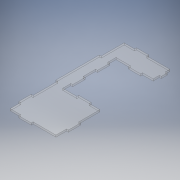
# Autodesk Inventor part: top
Saved by Autodesk Inventor 2017.2 (Build 212233000, 233)
## iProperties
Created: 2017-06-02
Part Number: top
Material: Polycarbonate, Clear
Document SubType Name: Modeling
Designer: SandeepSH
Density: 1.2 g/cm^3
Appearance: Polycarbonate - Clear
Author: SandeepSH
Autodesk Inventor part; units mm, degrees
ref_plane "YZ Plane" through (0, 0, 0) normal (1, 0, 0) x (0, 1, 0)
ref_plane "XZ Plane" through (0, 0, 0) normal (0, 1, 0) x (-1, 0, 0)
ref_plane "XY Plane" through (0, 0, 0) normal (0, 0, 1) x (1, 0, 0)
sketch "Sketch1" plane through (0, 0, 0) normal (0, 1, 0) x (-1, 0, 0)
  line L0 (-40, 95) -> (40, 95)
  line L1 (40, 95) -> (40, -95)
  line L2 (40, -95) -> (-40, -95)
  line L3 (-40, -95) -> (-40, 95)
  line L4 (-40, 95) -> (40, -95) construction
  line L5 (40, 95) -> (-40, -95) construction
  point P0 (0, 0)
  dimension "d0" = 80
  dimension "d1" = 190
  constraints: 12 end point, 2 midpoint, 2 parallel, 1 horizontal, 1 perpendicular
  measures "d0" distance of L1.end L2.end
  measures "d1" distance of L0.end L1.end
extrude "Extrusion1" add sketch "Sketch1" along normal blind 3
sketch "Sketch2" plane through (0, 3, 0) normal (0, 1, 0) x (1, 0, 0)
  line L0 (40, 95) -> (-40, 95) projected
  line L1 (-40, 95) -> (-37, 95)
  line L2 (-37, 95) -> (-37, 55)
  line L3 (-37, 55) -> (-40, 55)
  line L4 (-40, 55) -> (-40, 95)
  line L5 (-40, 95) -> (-40, -95) projected
  line L6 (-40, -95) -> (40, -95) projected
  line L7 (-37, 95) -> (-20, 95)
  line L8 (-20, 95) -> (-20, 92)
  line L9 (-20, 92) -> (-37, 92)
  line L10 (-37, 92) -> (-37, 95)
  line L11 (40, -95) -> (40, 95) projected
  line L12 (40, 95) -> (0, 95)
  line L13 (0, 95) -> (0, 92)
  line L14 (0, 92) -> (40, 92)
  line L15 (40, 92) -> (40, 95)
  line L16 (-40, -55) -> (-37, -55)
  line L17 (-37, -55) -> (-37, -15)
  line L18 (-37, -15) -> (-40, -15)
  line L19 (-40, -15) -> (-40, -55)
  line L20 (-40, -95) -> (-37, -95)
  line L21 (-37, -95) -> (-37, -75)
  line L22 (-37, -75) -> (-40, -75)
  line L23 (-40, -75) -> (-40, -95)
  line L24 (-37, -95) -> (-20, -95)
  line L25 (-20, -95) -> (-20, -92)
  line L26 (-20, -92) -> (-37, -92)
  line L27 (-37, -92) -> (-37, -95)
  line L28 (40, -95) -> (0, -95)
  line L29 (0, -95) -> (0, -92)
  line L30 (0, -92) -> (40, -92)
  line L31 (40, -92) -> (40, -95)
  line L32 (40, -18) -> (-20, -18)
  line L33 (-20, -18) -> (-20, 62)
  line L34 (-20, 62) -> (40, 62)
  line L35 (40, 62) -> (40, -18)
  line L36 (40, -92) -> (37, -92)
  line L37 (37, -92) -> (37, -75)
  line L38 (37, -75) -> (40, -75)
  line L39 (40, -75) -> (40, -92)
  line L40 (40, -18) -> (37, -18)
  line L41 (37, -18) -> (37, -55)
  line L42 (37, -55) -> (40, -55)
  line L43 (40, -55) -> (40, -18)
  line L44 (40, 92) -> (37, 92)
  line L45 (37, 92) -> (37, 85)
  line L46 (37, 85) -> (40, 85)
  line L47 (40, 85) -> (40, 92)
  line L48 (40, 62) -> (37, 62)
  line L49 (37, 62) -> (37, 75)
  line L50 (37, 75) -> (40, 75)
  line L51 (40, 75) -> (40, 62)
  line L52 (-20, -18) -> (-23, -18)
  line L53 (-23, -18) -> (-23, -8)
  line L54 (-23, -8) -> (-20, -8)
  line L55 (-20, -8) -> (-20, -18)
  line L56 (-20, 12) -> (-23, 12)
  line L57 (-23, 12) -> (-23, 32)
  line L58 (-23, 32) -> (-20, 32)
  line L59 (-20, 32) -> (-20, 12)
  line L60 (-20, 62) -> (-23, 62)
  line L61 (-23, 62) -> (-23, 52)
  line L62 (-23, 52) -> (-20, 52)
  line L63 (-20, 52) -> (-20, 62)
  line L64 (-23, -18) -> (0, -18)
  line L65 (0, -18) -> (0, -21)
  line L66 (0, -21) -> (-23, -21)
  line L67 (-23, -21) -> (-23, -18)
  line L68 (37, -18) -> (20, -18)
  line L69 (20, -18) -> (20, -21)
  line L70 (20, -21) -> (37, -21)
  line L71 (37, -21) -> (37, -18)
  line L72 (-23, 62) -> (0, 62)
  line L73 (0, 62) -> (0, 65)
  line L74 (0, 65) -> (-23, 65)
  line L75 (-23, 65) -> (-23, 62)
  line L76 (37, 62) -> (20, 62)
  line L77 (20, 62) -> (20, 65)
  line L78 (20, 65) -> (37, 65)
  line L79 (37, 65) -> (37, 62)
  point P0 (0, 0)
  dimension "d4" = 3
  dimension "d5" = 40
  dimension "d9" = 17
  dimension "d10" = 3
  dimension "d11" = 3
  dimension "d12" = 20
  dimension "d13" = 3
  dimension "d14" = 70
  dimension "d15" = 40
  dimension "d16" = 3
  dimension "d17" = 20
  dimension "d18" = 17
  dimension "d19" = 3
  dimension "d20" = 33
  dimension "d21" = 20
  dimension "d22" = 77
  dimension "d23" = 3
  dimension "d24" = 17
  dimension "d25" = 20
  dimension "d26" = 7
  dimension "d27" = 10
  dimension "d28" = 3
  dimension "d29" = 10
  dimension "d30" = 3
  dimension "d31" = 20
  dimension "d32" = 10
  dimension "d33" = 20
  dimension "d34" = 23
  dimension "d35" = 3
  dimension "d36" = 17
  dimension "d37" = 3
  dimension "d38" = 23
  dimension "d39" = 3
  dimension "d40" = 17
  dimension "d41" = 3
  constraints: 152 end point, 38 parallel, 19 horizontal, 19 perpendicular, 7 point on line
  measures "d4" distance of L2.end L3.end
  measures "d5" distance of L1.end L2.end
  measures "d9" distance of L8.end L9.end
  measures "d10" distance of L7.end L8.end
  measures "d11" distance of L13.end L12.end
  measures "d12" distance between parallel lines of L8 L13
  measures "d13" distance of L18.end L17.end
  measures "d14" distance between parallel lines of L3 L18
  measures "d15" distance between parallel lines of L16 L6
  measures "d16" distance of L22.end L21.end
  measures "d17" distance of L21.end L20.end
  measures "d18" distance of L26.end L25.end
  measures "d19" distance of L25.end L24.end
  measures "d20" distance between parallel lines of L0 L34
  measures "d21" distance between parallel lines of L5 L33
  measures "d22" distance between parallel lines of L6 L32
  measures "d23" distance of L37.end L38.end
  measures "d24" distance of L36.end L37.end
  measures "d25" distance between parallel lines of L42 L38
  measures "d26" distance of L45.end L44.end
  measures "d27" distance between parallel lines of L46 L50
  measures "d28" distance of L53.end L54.end
  measures "d29" distance of L52.end L53.end
  measures "d30" distance of L57.end L58.end
  measures "d31" distance of L56.end L57.end
  measures "d32" distance of L61.end L60.end
  measures "d33" distance between parallel lines of L56 L54
  measures "d34" distance of L65.end L66.end
  measures "d35" distance of L64.end L65.end
  measures "d36" distance of L70.end L69.end
  measures "d37" distance of L69.end L68.end
  measures "d38" distance of L74.end L73.end
  measures "d39" distance of L73.end L72.end
  measures "d40" distance of L77.end L78.end
  measures "d41" distance of L76.end L77.end
extrude "Extrusion2" cut sketch "Sketch2" against normal through all contours L11 L14 L13 L0 | L11 L46 L45 L14 | L8 L9 L2 L0 | L2 L3 L4 L0 | L11 L34 L49 L50 | L11 L32 L33 L34 | L11 L42 L41 L32 | L34 L77 L78 L49 | L18 L17 L16 L5 | L41 L70 L69 L32 | L11 L30 L37 L38 | L34 L60 L75 L74 L73 | L22 L21 L6 L5 | L11 L6 L29 L30 | L65 L66 L67 L52 L32 | L33 L62 L61 L60 | L52 L53 L54 L33 | L21 L26 L25 L6 | L33 L56 L57 L58
equation "\"d32\" = d29"
body "Solid1"
